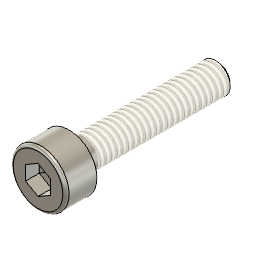
rpi_z2w_case (Autodesk Fusion 360 archive; units mm, degrees)
design "Hexagon Socket Head Cap Screw DIN 912 - M2.5 x 0.45 x 12 Steel 4.6 Plain"
description: Hexagon Socket Head Cap Screw DIN 912 - M2.5 x 0.45 x 12
part number: DIN 912 - M2.5 x 0.45 x 12 Steel 4.6 Plain
Autodesk Fusion 360 part; units mm, degrees
sketch "Sketch1" plane through (0, 0, 0) normal (0, 1, 0) x (1, 0, 0)
  line L0 (-1.25, 0) -> (-1.25, 12)
  line L1 (-1.25, 12) -> (0, 12)
  line L2 (0, 12) -> (0, -2.5)
  line L3 (-1.25, 0) -> (-2.25, 0)
  line L4 (-2.25, 0) -> (-2.25, -2.5)
  line L5 (-2.25, -2.5) -> (0, -2.5)
  dimension "d101" = 12
  dimension "d102" = 2.5
  dimension "d109" = 4.5
  dimension "d110" = 2.5
  constraint perpendicular L0 L1
  constraint collinear origin L1.end L2.end
  constraint perpendicular L0 L3
  constraint coincident origin L3
  constraint vertical L2
  constraint coincident L2 L5.end
  constraint perpendicular L2 L5
  measures "d101" distance of origin L1
  measures "d102" distance of L3.end L5
revolve "Revolve1" add sketch "Sketch1" angle 360 about axis through (0, 0, -12) along (0, 0, 1)
ref_plane "WorkPlane1" through (0, 0, 2.5) normal (0, 0, 1) x (1, 0, 0)
sketch "Sketch6" plane through (0, 0, 2.5) normal (0, 0, 1) x (1, 0, 0)
  line L0 (0, -1.1547) -> (1, -0.5774)
  line L1 (1, -0.5774) -> (1, 0.5774)
  line L2 (1, 0.5774) -> (0, 1.1547)
  line L3 (0, 1.1547) -> (-1, 0.5774)
  line L4 (-1, 0.5774) -> (-1, -0.5774)
  line L5 (-1, -0.5774) -> (0, -1.1547)
  dimension "d111" = 2
  constraint vertical L1
  measures "d111" distance of L1 L4
extrude "Extrude1" cut sketch "Sketch6" against normal blind 1.1
extrude "Extrude2" cut 1 faces at (-0.3333, -0.1925, 1.4) along direction (0, 0, -1) blind 1.1 draft -85
thread "Thread3" "ISO Metric profile 2.5 M2.5x0.45 M2.5x0.45 6g" major diameter 2.43 minor diameter 1.9165 pitch 0.45 angle 60 resizes the face on face at (-1.2438, 0.1245, -8) from (0, 0, -1.125) to (0, 0, -12)
fillet "Fillet4" radius 0.25 1 edges at (-2.0977, 0.8136, 2.5)
sketch "Sketch7" plane through (0, 0, 0) normal (0, 1, 0) x (1, 0, 0)
  line L0 (-1.275, 12) -> (-1.275, 11.7239)
  line L1 (-1.275, 11.7239) -> (-0.9739, 12)
  line L2 (0, 12) -> (0, -2.5)
  line L3 (-1.275, 12) -> (0, 12)
  dimension "d104" = 0.9739
  dimension "d105" = 1.275
  dimension "d106" = 0.2761
  constraint coincident L2.start L3.end
  constraint perpendicular L2 L3
  constraint coincident L1.end L3
  constraint perpendicular L0 L3
  measures "d104" distance of L1.end L2
  measures "d105" distance of L0 L2.start
  measures "d106" distance of L0.end L3
revolve "Revolve3" cut sketch "Sketch7" angle 360 about axis through (0, 0, 1.75) along (0, 0, 1)
equation "adsk_nomlen = 12.00 mm"
equation "adsk_headh = 2.50 mm"
equation "adsk_headdia = 4.50 mm"
equation "adsk_nomdia = 2.50 mm"
equation "adsk_philwidth = 2.00 mm"
equation "d31 = -adsk_phildepth"
equation "adsk_phildepth = 1.10 mm"
equation "d71 = adsk_headh"
equation "d76 = -adsk_phildepth"
equation "adsk_thrlen = 10.875 mm"
equation "d86 = adsk_nomdia * 0.1"
equation "adsk_startlen = 0.2760525 mm"
equation "adsk_endpointdia = 1.947895 mm"
equation "d101 = adsk_nomlen"
equation "d102 = adsk_headh"
equation "d104 = adsk_endpointdia / 2"
equation "d105 = adsk_nomdia * 0.51"
equation "d106 = adsk_startlen"
equation "d108 = min(adsk_thrlen; adsk_nomlen - 0.001 mm)"
equation "d109 = adsk_headdia"
equation "d110 = adsk_nomdia"
equation "d111 = adsk_philwidth"

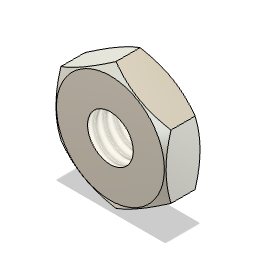
design "Hexagon Nut BS 4183 - M2.5 Steel 6 Plain"
description: Hexagon Nut BS 4183 - M2.5
part number: HN BS 4183 - M2.5 Steel 6 Plain
Autodesk Fusion 360 part; units mm, degrees
sketch "Sketch1" plane through (0, 0, 0) normal (0, 1, 0) x (1, 0, 0)
  line L0 (0, 0) -> (0, -1.6)
  line L1 (-1.25, 0) -> (-2.45, 0)
  line L2 (-2.45, 0) -> (-2.8875, -0.2526)
  line L3 (-2.8875, -0.2526) -> (-2.8875, -1.3474)
  line L4 (-2.8875, -1.3474) -> (-2.45, -1.6)
  line L5 (-2.45, -1.6) -> (-1.25, -1.6)
  line L6 (-1.25, -1.6) -> (-1.25, 0)
  dimension "d121" = 2.5
  dimension "d122" = 30
  dimension "d123" = 30
  dimension "d125" = 4.9
  dimension "d128" = 5.775
  dimension "d152" = 1.6
  constraint vertical L0
  constraint coincident L0 L0.end
  constraint coincident origin L0
  constraint horizontal L1
  constraint perpendicular L1 L3
  constraint perpendicular L3 L5
  constraint perpendicular L5 L6
  constraint coincident L0.start L1
  constraint coincident L0.start origin
  constraint vertical L1.end L4.end
  constraint coincident L0.end L5
  measures "d122" angle of L1 L2
  measures "d123" angle of L4 L5
  measures "d152" distance of L1.start L5
revolve "Revolve1" add sketch "Sketch1" angle 360 about axis through (0, 0, 0) along (0, 0, 1)
sketch "Sketch8" plane through (0, 0, 1.6) normal (0, 0, 1) x (1, 0, 0)
  line L0 (0, 0) -> (-5, 0) construction
  line L1 (-2.5, -1.4449) -> (-2.5, 1.4449)
  circle A0 centre (0, 0) radius 1.25
  circle A1 centre (0, 0) radius 2.8875
  dimension "d114" = 2.5
  constraint horizontal L0
  constraint perpendicular L0 L1
  constraint midpoint L0 L1
  constraint coincident L0.start A0.centre
  constraint coincident L1.end A1
  measures "d114" distance of L0.start L1
extrude "Extrude5" cut sketch "Sketch8" against normal blind 1.6 contours L1 A1 picked at (-2.5625, 0.3519)
pattern_circular "C-Pattern2" count 6 over 360 about axis through (0, 0, 1.75) along (0, 0, 1) of "Extrude5"
thread "Thread3" "ISO Metric profile 2.5 M2.5x0.45 M2.5x0.45 6H" major diameter 2.58 minor diameter 2.0755 pitch 0.45 angle 60 resizes the face on face at (-1.2484, 0.0623, 1.0667)
equation "adsk_nheig = 1.60 mm"
equation "adsk_maxdia = 5.775 mm"
equation "adsk_nomdia = 2.50 mm"
equation "d89 = -adsk_nheig"
equation "adsk_waflat = 5.00 mm"
equation "d114 = adsk_waflat / 2"
equation "adsk_chamang1 = 30 deg"
equation "adsk_chamang2 = 30 deg"
equation "d121 = adsk_nomdia"
equation "d122 = adsk_chamang1"
equation "d123 = adsk_chamang2"
equation "d125 = adsk_beardia"
equation "d128 = adsk_maxdia"
equation "d147 = adsk_nheig"
equation "adsk_beardia = adsk_waflat * 0.98"
equation "d152 = adsk_nheig"
